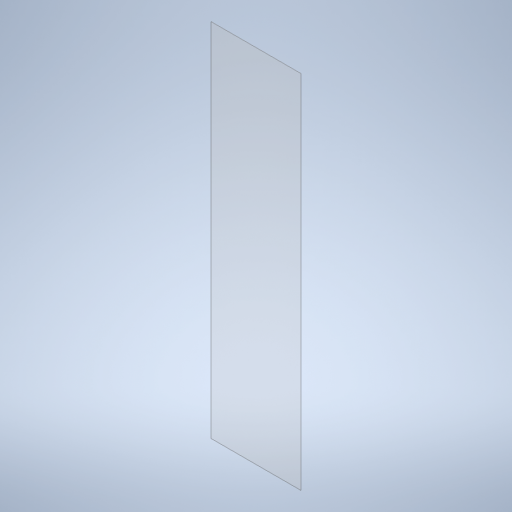
# Autodesk Inventor part: Window
Saved by Autodesk Inventor 2023.1 (Build 271208000, 208)
## iProperties
Created: 2023-06-06
Part Number: Window
Material: Polycarbonate, Clear
Document SubType Name: Modeling
Designer: rwc6
Density: 1.2 g/cm^3
Appearance: Polycarbonate - Clear
win_d: 0.006 m
win_h: 4.900 m
win_w: 1.219 m
Author: rwc6
Autodesk Inventor part; units mm, degrees
ref_plane "YZ Plane" through (0, 0, 0) normal (1, 0, 0) x (0, 1, 0)
ref_plane "XZ Plane" through (0, 0, 0) normal (0, 1, 0) x (-1, 0, 0)
ref_plane "XY Plane" through (0, 0, 0) normal (0, 0, 1) x (1, 0, 0)
sketch "Sketch1" plane through (0, 0, 0) normal (0, 0, 1) x (1, 0, 0)
  line L0 (-609.6, -2450) -> (609.6, -2450)
  line L1 (609.6, -2450) -> (609.6, 2450)
  line L2 (609.6, 2450) -> (-609.6, 2450)
  line L3 (-609.6, 2450) -> (-609.6, -2450)
  line L4 (-609.6, -2450) -> (609.6, 2450) construction
  line L5 (609.6, -2450) -> (-609.6, 2450) construction
  point P0 (0, 0)
  dimension "d0" = 1219.2
  dimension "d1" = 4900
  constraints: 12 end point, 2 midpoint, 2 parallel, 1 horizontal, 1 perpendicular
  measures "d0" distance of L2.end L1.end
  measures "d1" distance of L1.end L0.end
extrude "Extrusion1" add sketch "Sketch1" along normal mid plane 6.4
equation "\"d0\" = win_w"
equation "\"d1\" = win_h"
equation "\"d2\" = win_d"
equation "\"win_h\" = 4900"
equation "\"win_w\" = 1219.2"
equation "\"win_d\" = 6.4"
